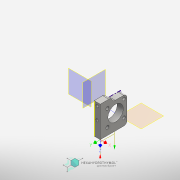
# Autodesk Inventor part: C-head-base
Saved by Autodesk Inventor 2016 (Build 200138000, 138)
## iProperties
Created: 2015-05-08
Part Number: C-head-base
Material: Generic
Document SubType Name: Modeling
Designer: ax
Density: 1 g/cm^3
Appearance: Default
Mass: 2.92984 g
Surface Area: 24.0319 cm^2
Volume: 2.92984 cm^3
cMotorSize: 30.000 mm
d1: 30.000 mm
d4: 6,000 mm
d5: 30.000 mm
d6: 30.000 mm
d7: 0,00 deg
d16: 22.000 mm
d32: 15.000 mm
Author: ax
Autodesk Inventor part; units mm, degrees
ref_plane "YZ Plane" through (0, 0, 0) normal (1, 0, 0) x (0, 1, 0)
ref_plane "XZ Plane" through (0, 0, 0) normal (0, 1, 0) x (-1, 0, 0)
ref_plane "XY Plane" through (0, 0, 0) normal (0, 0, 1) x (1, 0, 0)
ref_plane "Work Plane3" through (0, 0, 6) normal (0, 0, 1) x (1, 0, 0)
sketch "Sketch2" plane through (0, 0, 6) normal (0, 0, 1) x (1, 0, 0)
  line L0 (0, -10) -> (-6, -10)
  line L1 (-6, -10) -> (-6, -40)
  line L2 (-6, -40) -> (0, -40)
  line L3 (0, -40) -> (0, -10)
  line L4 (0, -40) -> (-66, -40)
  line L5 (0, -40) -> (-66, -40) projected
  dimension "d4" = 6
  dimension "d5" = 30
  dimension "d83" = 0
  dimension "d84" = 0
  constraints: 10 end point, 3 perpendicular
  measures "d4" distance of L2.end L1.end
  measures "d5" distance of L1.end L0.end
  measures "d83" distance between parallel lines of L4 L2
  measures "d84" distance between parallel lines of L2 L5
extrude "Extrusion2" add sketch "Sketch2" along normal blind 30
ref_plane "Work Plane4" through (-60, 0, 0) normal (0, 1, 0) x (1, 0, 0)
ref_plane "Work Plane5" through (-6, -40, 46) normal (-1, 0, 0) x (0, 0, 1)
sketch "Sketch5" plane through (-6, -40, 46) normal (-1, 0, 0) x (0, 0, 1)
  line L0 (-36, 26) -> (-14, 26)
  line L1 (-14, 26) -> (-14, 4)
  line L2 (-14, 4) -> (-36, 4)
  line L3 (-36, 4) -> (-36, 26)
  line L4 (-36, 26) -> (-14, 4) construction
  line L5 (-14, 26) -> (-36, 4) construction
  line L6 (-40, 30) -> (-40, 0) projected
  line L7 (-40, 0) -> (-10, 0) projected
  point P0 (-25, 15)
  dimension "d16" = 22
  dimension "d85" = 15
  dimension "d86" = 15
  constraints: 12 end point, 2 midpoint, 2 parallel, 2 perpendicular, 1 coincident, 1 horizontal
  measures "d16" distance of L0.end L1.end
  measures "d85" distance from line of L6 point (-25, 15)
  measures "d86" distance from line of L7 point (-25, 15)
hole "Hole2" at (-6, -25, 21) direction (1, 0, 0) diameter 15 end through all
sketch "Sketch6" plane through (-6, -40, 6) normal (0, -1, 0) x (1, 0, 0)
  line L0 (0, 0) -> (6, 0) projected
  line L1 (6, 0) -> (6, 30) projected
  point P0 (3, 27)
  point P1 (3, 15)
  dimension "d47" = 27
  dimension "d48" = 15
  dimension "d49" = 3
  dimension "d50" = 3
  measures "d47" distance from line of L0 point (3, 27)
  measures "d48" distance from line of L0 point (3, 15)
  measures "d49" distance from line of L1 point (3, 15)
  measures "d50" distance from line of L1 point (3, 27)
hole "Hole3" at (-3, -40, 21) at (-3, -40, 33) direction (0, 1, 0) diameter 2.459 depth 8.8 tip angle 118 thread size "M3x0.5" class "6H" standard "ISO Metric profile"
sketch "Sketch7" plane through (-6, -40, 6) normal (0, -1, 0) x (1, 0, 0)
  point P0 (3, 15)
  point P1 (3, 27)
sketch "Sketch8" plane through (0, 0, 6) normal (0, 0, -1) x (-1, 0, 0)
  point P0 (3, -23)
  point P1 (3, -37)
hole "Hole5" at (-3, -23, 6) at (-3, -37, 6) direction (0, 0, 1) diameter 2.459 depth 7 tip angle 120 thread size "M3x0.5" class "6H" standard "ISO Metric profile"
sketch "Sketch9" plane through (-6, -40, 6) normal (-1, 0, 0) x (0, 0, 1)
  line L0 (23, 23) -> (7, 23)
  line L1 (7, 23) -> (7, 7)
  line L2 (7, 7) -> (23, 7)
  line L3 (23, 7) -> (23, 23)
  line L4 (23, 23) -> (7, 7) construction
  line L5 (7, 23) -> (23, 7) construction
  point P0 (-6, 40)
  point P1 (15, 15)
  dimension "d94" = 16
  dimension "d95" = 16
  constraints: 12 end point, 2 midpoint, 2 parallel, 1 horizontal, 1 perpendicular
  measures "d94" distance of L2.end L1.end
  measures "d95" distance of L1.end L0.end
hole "Hole8" at (-6, -33, 29) at (-6, -33, 13) at (-6, -17, 13) at (-6, -17, 29) direction (1, 0, 0) diameter 3 depth 8 tip angle 118
move faces "Move1" translate (0, -4, 0) faces at (-2, -10, 16)
sketch "Sketch10" plane through (-6, -40, 6) normal (-1, 0, 0) x (0, 0, 1)
  line L0 (0, 0) -> (30, 0) projected
  line L1 (30, 0) -> (30, 10)
  line L2 (30, 26) -> (30, 0) projected
  line L3 (30, 10) -> (26, 13)
  line L4 (26, 13) -> (26, 26)
  line L5 (0, 26) -> (30, 26) projected
  line L6 (30, 26) -> (30, 10)
  point P0 (-6, 40)
  dimension "d109" = 10
  constraints: 8 end point, 2 point on line, 1 collinear, 1 parallel
  measures "d109" distance of L0.end L1.end
extrude "Extrusion4" cut sketch "Sketch10" against normal blind 10
fillet "Fillet2" radius 3.1 4 edges at (-3, -27, 32) (-3, -30, 36) (-3, -14, 32) (-3, -14, 6)
equation "\"d5\" = d1"
equation "\"d6\" = cMotorSize"
equation "\"d85\" = 0.5 * cMotorSize"
equation "\"d86\" = 0.5 * cMotorSize"
equation "\"d48\" = 0.5 * cMotorSize"
equation "\"d50\" = d49"
equation "\"d1\" = cMotorSize"
equation "\"cMotorSize\" = 30"
body "Solid1"
